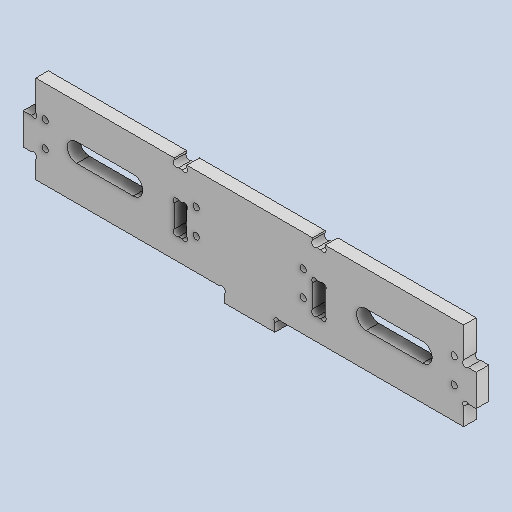
# Autodesk Inventor part: Inner Front Wall
Saved by Autodesk Inventor 2023 (Build 270158000, 158)
## iProperties
Created: 2022-12-26
Part Number: Inner Front Wall
Material: Generic
Document SubType Name: Modeling
Designer: justi
Density: 1 g/cm^3
Appearance: Default
Mass: 489.127 g
Surface Area: 960.562 cm^2
Volume: 489.127 cm^3
Author: justi
Autodesk Inventor part; units mm, degrees
ref_plane "YZ Plane" through (0, 0, 0) normal (1, 0, 0) x (0, 1, 0)
ref_plane "XZ Plane" through (0, 0, 0) normal (0, 1, 0) x (-1, 0, 0)
ref_plane "XY Plane" through (0, 0, 0) normal (0, 0, 1) x (1, 0, 0)
sketch "Sketch1" plane through (0, 0, 0) normal (0, 0, 1) x (1, 0, 0)
  line L0 (0, 0) -> (457.2, 0)
  line L1 (457.2, 0) -> (457.2, 101.6)
  line L2 (457.2, 101.6) -> (0, 101.6)
  line L3 (0, 101.6) -> (0, 0)
  line L4 (0, 101.6) -> (12.7, 101.6)
  line L5 (12.7, 101.6) -> (12.7, 66.675)
  line L6 (12.7, 66.675) -> (0, 66.675)
  line L7 (0, 66.675) -> (0, 101.6)
  line L8 (457.2, 101.6) -> (444.5, 101.6)
  line L9 (444.5, 101.6) -> (444.5, 66.675)
  line L10 (444.5, 66.675) -> (457.2, 66.675)
  line L11 (457.2, 66.675) -> (457.2, 101.6)
  line L12 (0, 0) -> (12.7, 0)
  line L13 (12.7, 0) -> (12.7, 34.925)
  line L14 (12.7, 34.925) -> (0, 34.925)
  line L15 (0, 34.925) -> (0, 0)
  line L16 (457.2, 0) -> (444.5, 0)
  line L17 (444.5, 0) -> (444.5, 34.925)
  line L18 (444.5, 34.925) -> (457.2, 34.925)
  line L19 (457.2, 34.925) -> (457.2, 0)
  line L20 (152.4, 101.6) -> (165.1, 101.6)
  line L21 (165.1, 101.6) -> (165.1, 95.25)
  line L22 (165.1, 95.25) -> (152.4, 95.25)
  line L23 (152.4, 95.25) -> (152.4, 101.6)
  line L24 (304.8, 101.6) -> (292.1, 101.6)
  line L25 (292.1, 101.6) -> (292.1, 95.25)
  line L26 (292.1, 95.25) -> (304.8, 95.25)
  line L27 (304.8, 95.25) -> (304.8, 101.6)
  line L28 (152.4, 66.675) -> (165.1, 66.675)
  line L29 (165.1, 66.675) -> (165.1, 34.925)
  line L30 (165.1, 34.925) -> (152.4, 34.925)
  line L31 (152.4, 34.925) -> (152.4, 66.675)
  line L32 (292.1, 66.675) -> (304.8, 66.675)
  line L33 (304.8, 66.675) -> (304.8, 34.925)
  line L34 (304.8, 34.925) -> (292.1, 34.925)
  line L35 (292.1, 34.925) -> (292.1, 66.675)
  line L36 (12.7, 0) -> (203.2, 0)
  line L37 (203.2, 0) -> (203.2, 12.7)
  line L38 (203.2, 12.7) -> (12.7, 12.7)
  line L39 (12.7, 12.7) -> (12.7, 0)
  line L40 (444.5, 0) -> (254, 0)
  line L41 (254, 0) -> (254, 12.7)
  line L42 (254, 12.7) -> (444.5, 12.7)
  line L43 (444.5, 12.7) -> (444.5, 0)
  point P0 (0, 66.675)
  point P1 (12.7, 12.7)
  point P2 (292.1, 101.6)
  point P3 (165.1, 101.6)
  dimension "d0" = 101.6
  dimension "d1" = 457.2
  dimension "d2" = 12.7
  dimension "d3" = 34.925
  dimension "d4" = 12.7
  dimension "d5" = 34.925
  dimension "d6" = 12.7
  dimension "d7" = 34.925
  dimension "d8" = 12.7
  dimension "d9" = 34.925
  dimension "d13" = 12.7
  dimension "d14" = 6.35
  dimension "d15" = 139.7
  dimension "d16" = 12.7
  dimension "d17" = 6.35
  dimension "d18" = 139.7
  dimension "d19" = 12.7
  dimension "d20" = 139.7
  dimension "d21" = 28.575
  dimension "d22" = 12.7
  dimension "d23" = 139.7
  dimension "d24" = 28.575
  dimension "d25" = 31.75
  dimension "d26" = 31.75
  dimension "d27" = 190.5
  dimension "d28" = 12.7
  dimension "d29" = 190.5
  dimension "d30" = 12.7
  constraints: 88 end point, 22 parallel, 11 horizontal, 11 perpendicular, 2 point on line
  measures "d0" distance of L0.end L1.end
  measures "d1" distance of L1.end L2.end
  measures "d2" distance of L5.end L6.end
  measures "d3" distance of L4.end L5.end
  measures "d4" distance of L10.end L9.end
  measures "d5" distance of L8.end L9.end
  measures "d6" distance of L14.end L13.end
  measures "d7" distance of L12.end L13.end
  measures "d8" distance of L17.end L18.end
  measures "d9" distance of L16.end L17.end
  measures "d13" distance of L21.end L22.end
  measures "d14" distance of L22.end L20.start
  measures "d15" distance between parallel lines of L5 L23
  measures "d16" distance of L26.end L25.end
  measures "d17" distance of L24.end L25.end
  measures "d18" distance between parallel lines of L9 L27
  measures "d19" distance of L29.end L30.end
  measures "d20" distance between parallel lines of L5 L31
  measures "d21" distance between parallel lines of L22 L28
  measures "d22" distance of L33.end L34.end
  measures "d23" distance between parallel lines of L9 L33
  measures "d24" distance between parallel lines of L26 L32
  measures "d25" distance of L28.end L29.end
  measures "d26" distance of L34.end L32.start
  measures "d27" distance of L38.end L37.end
  measures "d28" distance of L36.end L37.end
  measures "d29" distance of L41.end L42.end
  measures "d30" distance of L40.end L41.end
extrude "Extrusion1" add sketch "Sketch1" along normal blind 12.7 contours L3 L6 L5 L2 L23 L22 L21 L25 L26 L27 L9 L10 L1 L18 L17 L42 L41 L0 L37 L38 L13 L14
sketch "Sketch3" plane through (0, 0, 12.7) normal (0, 0, 1) x (1, 0, 0)
  line L0 (12.7, 101.6) -> (12.7, 66.675) projected
  line L1 (12.7, 66.675) -> (10.4549, 68.9201)
  circle A0 centre (10.4549, 68.9201) radius 3.175
  line L2 (12.7, 34.925) -> (12.7, 12.7) projected
  line L3 (12.7, 34.925) -> (10.4549, 32.6799)
  circle A1 centre (10.4549, 32.6799) radius 3.175
  line L4 (203.2, 12.7) -> (203.2, 0) projected
  line L5 (203.2, 12.7) -> (200.9549, 10.4549)
  circle A2 centre (200.9549, 10.4549) radius 3.175
  line L6 (254, 0) -> (254, 12.7) projected
  line L7 (254, 12.7) -> (256.2451, 10.4549)
  line L8 (254, 12.7) -> (444.5, 12.7) projected
  circle A3 centre (256.2451, 10.4549) radius 3.175
  line L9 (444.5, 34.925) -> (446.7451, 32.6799)
  line L10 (444.5, 34.925) -> (457.2, 34.925) projected
  circle A4 centre (446.7451, 32.6799) radius 3.175
  line L11 (457.2, 66.675) -> (444.5, 66.675) projected
  line L12 (444.5, 66.675) -> (446.7451, 68.9201)
  circle A5 centre (446.7451, 68.9201) radius 3.175
  line L13 (304.8, 34.925) -> (292.1, 34.925) projected
  line L14 (292.1, 34.925) -> (294.3451, 37.1701)
  line L15 (304.8, 34.925) -> (302.5549, 37.1701)
  line L16 (304.8, 66.675) -> (304.8, 34.925) projected
  line L17 (292.1, 66.675) -> (304.8, 66.675) projected
  line L18 (292.1, 66.675) -> (294.3451, 64.4299)
  line L19 (304.8, 66.675) -> (302.5549, 64.4299)
  line L20 (304.8, 95.25) -> (292.1, 95.25) projected
  line L21 (292.1, 95.25) -> (294.3451, 97.4951)
  line L22 (304.8, 95.25) -> (302.5549, 97.4951)
  line L23 (304.8, 101.6) -> (304.8, 95.25) projected
  line L24 (165.1, 34.925) -> (152.4, 34.925) projected
  line L25 (152.4, 34.925) -> (154.6451, 37.1701)
  line L26 (165.1, 66.675) -> (165.1, 34.925) projected
  line L27 (165.1, 34.925) -> (162.8549, 37.1701)
  line L28 (152.4, 66.675) -> (165.1, 66.675) projected
  line L29 (152.4, 66.675) -> (154.6451, 64.4299)
  line L30 (165.1, 66.675) -> (162.8549, 64.4299)
  line L31 (165.1, 95.25) -> (152.4, 95.25) projected
  line L32 (152.4, 95.25) -> (154.6451, 97.4951)
  line L33 (165.1, 95.25) -> (162.8549, 97.4951)
  line L34 (165.1, 101.6) -> (165.1, 95.25) projected
  circle A6 centre (154.6451, 97.4951) radius 3.175
  circle A7 centre (162.8549, 97.4951) radius 3.175
  circle A8 centre (154.6451, 64.4299) radius 3.175
  circle A9 centre (162.8549, 64.4299) radius 3.175
  circle A10 centre (162.8549, 37.1701) radius 3.175
  circle A11 centre (154.6451, 37.1701) radius 3.175
  circle A12 centre (294.3451, 37.1701) radius 3.175
  circle A13 centre (302.5549, 37.1701) radius 3.175
  circle A14 centre (294.3451, 64.4299) radius 3.175
  circle A15 centre (302.5549, 64.4299) radius 3.175
  circle A16 centre (294.3451, 97.4951) radius 3.175
  circle A17 centre (302.5549, 97.4951) radius 3.175
  point P0 (0, 0)
  dimension "d38" = 3.175
  dimension "d39" = 45
  dimension "d40" = 6.35
  dimension "d41" = 3.175
  dimension "d42" = 45
  dimension "d43" = 6.35
  dimension "d44" = 3.175
  dimension "d45" = 45
  dimension "d46" = 6.35
  dimension "d47" = 3.175
  dimension "d48" = 45
  dimension "d49" = 6.35
  dimension "d50" = 3.175
  dimension "d51" = 45
  dimension "d52" = 6.35
  dimension "d53" = 3.175
  dimension "d54" = 45
  dimension "d55" = 6.35
  dimension "d56" = 3.175
  dimension "d57" = 45
  dimension "d58" = 3.175
  dimension "d59" = 45
  dimension "d60" = 3.175
  dimension "d61" = 45
  dimension "d62" = 3.175
  dimension "d63" = 45
  dimension "d64" = 3.175
  dimension "d65" = 45
  dimension "d66" = 3.175
  dimension "d67" = 45
  dimension "d68" = 3.175
  dimension "d69" = 45
  dimension "d70" = 3.175
  dimension "d71" = 45
  dimension "d72" = 3.175
  dimension "d73" = 45
  dimension "d74" = 3.175
  dimension "d75" = 45
  dimension "d76" = 3.175
  dimension "d77" = 45
  dimension "d78" = 3.175
  dimension "d79" = 45
  dimension "d80" = 6.35
  dimension "d81" = 6.35
  dimension "d82" = 6.35
  dimension "d83" = 6.35
  dimension "d84" = 6.35
  dimension "d85" = 6.35
  dimension "d86" = 6.35
  dimension "d87" = 6.35
  dimension "d88" = 6.35
  dimension "d89" = 6.35
  dimension "d90" = 6.35
  dimension "d91" = 6.35
  constraints: 36 end point, 18 centre point, 14 point on line, 2 coincident
  measures "d38" distance of L0.end L1.end
  measures "d39" angle of L0 L1
  measures "d40" diameter of A0
  measures "d41" distance of L2.start L3.end
  measures "d42" angle of L2 L3
  measures "d43" diameter of A1
  measures "d44" distance of L4.start L5.end
  measures "d45" angle of L4 L5
  measures "d46" diameter of A2
  measures "d47" distance of L6.end L7.end
  measures "d48" angle of L8 L7
  measures "d49" diameter of A3
  measures "d50" distance of L9.start L9.end
  measures "d51" angle of L10 L9
  measures "d52" diameter of A4
  measures "d53" distance of L11.end L12.end
  measures "d54" angle of L11 L12
  measures "d55" diameter of A5
  measures "d56" distance of L13.end L14.end
  measures "d57" angle of L13 L14
  measures "d58" distance of L13.start L15.end
  measures "d59" angle of L16 L15
  measures "d60" distance of L17.start L18.end
  measures "d61" angle of L17 L18
  measures "d62" distance of L16.start L19.end
  measures "d63" angle of L16 L19
  measures "d64" distance of L20.end L21.end
  measures "d65" angle of L20 L21
  measures "d66" distance of L20.start L22.end
  measures "d67" angle of L23 L22
  measures "d68" distance of L24.end L25.end
  measures "d69" angle of L24 L25
  measures "d70" distance of L24.start L27.end
  measures "d71" angle of L26 L27
  measures "d72" distance of L28.start L29.end
  measures "d73" angle of L28 L29
  measures "d74" distance of L26.start L30.end
  measures "d75" angle of L26 L30
  measures "d76" distance of L31.end L32.end
  measures "d77" angle of L31 L32
  measures "d78" distance of L31.start L33.end
  measures "d79" angle of L34 L33
  measures "d80" diameter of A6
  measures "d81" diameter of A7
  measures "d82" diameter of A8
  measures "d83" diameter of A9
  measures "d84" diameter of A10
  measures "d85" diameter of A11
  measures "d86" diameter of A12
  measures "d87" diameter of A13
  measures "d88" diameter of A14
  measures "d89" diameter of A15
  measures "d90" diameter of A16
  measures "d91" diameter of A17
extrude "Extrusion3" cut sketch "Sketch3" against normal blind 25.4
sketch "Sketch6" plane through (0, 0, 12.7) normal (0, 0, 1) x (1, 0, 0)
  circle A0 centre (22.225, 69.85) radius 3.175
  line L0 (152.4, 101.6) -> (12.7, 101.6) projected
  line L1 (12.7, 101.6) -> (12.7, 71.1651) projected
  circle A1 centre (174.625, 69.85) radius 3.175
  line L2 (292.1, 101.6) -> (165.1, 101.6) projected
  line L3 (165.1, 62.1849) -> (165.1, 39.4151) projected
  circle A2 centre (282.575, 69.85) radius 3.175
  line L4 (292.1, 39.4151) -> (292.1, 62.1849) projected
  circle A3 centre (282.575, 44.45) radius 3.175
  circle A4 centre (174.625, 44.45) radius 3.175
  circle A5 centre (22.225, 44.45) radius 3.175
  circle A6 centre (434.975, 69.85) radius 3.175
  line L5 (444.5, 101.6) -> (304.8, 101.6) projected
  line L6 (444.5, 71.1651) -> (444.5, 101.6) projected
  circle A7 centre (434.975, 44.45) radius 3.175
  line L7 (444.5, 12.7) -> (444.5, 30.4349) projected
  point P0 (0, 0)
  dimension "d146" = 6.35
  dimension "d147" = 31.75
  dimension "d148" = 9.525
  dimension "d149" = 6.35
  dimension "d150" = 31.75
  dimension "d151" = 9.525
  dimension "d152" = 6.35
  dimension "d153" = 31.75
  dimension "d154" = 9.525
  dimension "d155" = 6.35
  dimension "d156" = 9.525
  dimension "d157" = 25.4
  dimension "d158" = 6.35
  dimension "d159" = 9.525
  dimension "d160" = 25.4
  dimension "d161" = 6.35
  dimension "d162" = 9.525
  dimension "d163" = 25.4
  dimension "d164" = 6.35
  dimension "d165" = 31.75
  dimension "d166" = 9.525
  dimension "d167" = 6.35
  dimension "d168" = 9.525
  dimension "d169" = 25.4
  constraints: 8 centre point
  measures "d146" diameter of A0
  measures "d147" distance from line of L0 A0.centre
  measures "d148" distance from line of L1 A0.centre
  measures "d149" diameter of A1
  measures "d150" distance from line of L2 A1.centre
  measures "d151" distance from line of L3 A1.centre
  measures "d152" diameter of A2
  measures "d153" distance from line of L2 A2.centre
  measures "d154" distance from line of L4 A2.centre
  measures "d155" diameter of A3
  measures "d156" distance from line of L4 A3.centre
  measures "d157" distance of A2.centre A3.centre
  measures "d158" diameter of A4
  measures "d159" distance from line of L3 A4.centre
  measures "d160" distance of A1.centre A4.centre
  measures "d161" diameter of A5
  measures "d162" distance from line of L1 A5.centre
  measures "d163" distance of A0.centre A5.centre
  measures "d164" diameter of A6
  measures "d165" distance from line of L5 A6.centre
  measures "d166" distance from line of L6 A6.centre
  measures "d167" diameter of A7
  measures "d168" distance from line of L7 A7.centre
  measures "d169" distance of A6.centre A7.centre
extrude "Extrusion5" cut sketch "Sketch6" against normal blind 12.7
sketch "Sketch7" plane through (0, 0, 12.7) normal (0, 0, 1) x (1, 0, 0)
  line L0 (44.45, 66.675) -> (120.65, 66.675)
  line L1 (120.65, 66.675) -> (120.65, 47.625)
  line L2 (120.65, 47.625) -> (44.45, 47.625)
  line L3 (44.45, 47.625) -> (44.45, 66.675)
  line L4 (12.7, 101.6) -> (12.7, 71.1651) projected
  line L5 (152.4, 101.6) -> (12.7, 101.6) projected
  line L6 (336.55, 66.675) -> (412.75, 66.675)
  line L7 (412.75, 66.675) -> (412.75, 47.625)
  line L8 (412.75, 47.625) -> (336.55, 47.625)
  line L9 (336.55, 47.625) -> (336.55, 66.675)
  line L10 (444.5, 101.6) -> (304.8, 101.6) projected
  line L11 (444.5, 12.7) -> (444.5, 30.4349) projected
  point P0 (0, 0)
  point P1 (82.55, 66.675)
  point P2 (44.45, 57.15)
  point P3 (412.75, 57.15)
  point P4 (374.65, 66.675)
  dimension "d172" = 19.05
  dimension "d173" = 76.2
  dimension "d174" = 69.85
  dimension "d175" = 44.45
  dimension "d176" = 76.2
  dimension "d177" = 19.05
  dimension "d178" = 44.45
  dimension "d179" = 69.85
  constraints: 16 end point, 4 midpoint, 4 parallel, 2 horizontal, 2 perpendicular
  measures "d172" distance of L0.end L1.end
  measures "d173" distance of L0.start L0.end
  measures "d174" distance from line of L4 point (82.55, 66.675)
  measures "d175" distance from line of L5 point (44.45, 57.15)
  measures "d176" distance of L6.start L6.end
  measures "d177" distance of L6.end L7.end
  measures "d178" distance from line of L10 point (412.75, 57.15)
  measures "d179" distance from line of L11 point (374.65, 66.675)
extrude "Extrusion6" cut sketch "Sketch7" against normal blind 12.7
fillet "Fillet1" radius 9.525 8 edges at (44.45, 47.625, 6.35) (44.45, 66.675, 6.35) (120.65, 66.675, 6.35) (120.65, 47.625, 6.35) (336.55, 66.675, 6.35) (336.55, 47.625, 6.35) (412.75, 47.625, 6.35) (412.75, 66.675, 6.35)
body "Solid1"
